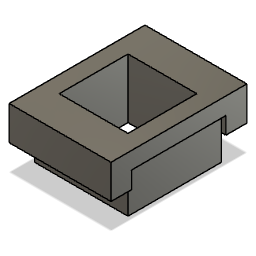
switch_holder (Autodesk Fusion 360 design; units mm, degrees)
Autodesk Fusion 360 part; units mm, degrees
note: some values were not read from the file. Set by a fixed rule: which sketch regions a step uses.
sketch "Sketch1" plane through (0, 0, 0) normal (0, 1, 0) x (1, 0, 0)
  line L0 (5.5, 5.5) -> (-5.5, 5.5)
  line L1 (-5.5, 5.5) -> (-5.5, -5.5)
  line L2 (-5.5, -5.5) -> (5.5, -5.5)
  line L3 (5.5, -5.5) -> (5.5, 5.5)
  line L4 (5.5, 5.5) -> (-5.5, -5.5) construction
  line L5 (-5.5, 5.5) -> (5.5, -5.5) construction
  dimension "d1" = 11
  dimension "d2" = 11
  constraint horizontal L0
  constraint perpendicular L0 L1
  constraint parallel L0 L2
  constraint parallel L1 L3
  constraint coincident L4 origin
  constraint coincident L5 origin
  measures "d1" distance of L1.end L2.end
  measures "d2" distance of L0.end L1.end
extrude "Extrude1" add sketch "Sketch1" along normal blind 5
sketch "Sketch2" plane through (0, 5, 0) normal (0, 1, 0) x (-1, 0, 0)
  line L0 (-5.5, 5.5) -> (-5.5, -5.5)
  line L1 (-5.5, -5.5) -> (5.5, -5.5)
  line L2 (5.5, -5.5) -> (5.5, 5.5)
  line L3 (5.5, 5.5) -> (-5.5, 5.5)
  line L4 (-4.05, -4.05) -> (4.05, -4.05)
  line L5 (4.05, -4.05) -> (4.05, 4.05)
  line L6 (4.05, 4.05) -> (-4.05, 4.05)
  line L7 (-4.05, 4.05) -> (-4.05, -4.05)
  line L8 (-4.05, -4.05) -> (4.05, 4.05) construction
  line L9 (4.05, -4.05) -> (-4.05, 4.05) construction
  dimension "d5" = 8.1
  dimension "d6" = 8.1
  constraint horizontal L4
  constraint perpendicular L4 L5
  constraint parallel L4 L6
  constraint parallel L5 L7
  constraint coincident L8 origin
  constraint coincident L9 origin
  measures "d5" distance of L5.end L6.end
  measures "d6" distance of L4.end L5.end
extrude "Extrude2" cut sketch "Sketch2" against normal blind 5 contours L4 L5 L6 L7
sketch "Sketch3" plane through (0, 5, 0) normal (0, 1, 0) x (-1, 0, 0)
  line L0 (4.05, -4.05) -> (-4.05, -4.05)
  line L1 (-4.05, -4.05) -> (-4.05, 4.05)
  line L2 (-4.05, 4.05) -> (4.05, 4.05)
  line L3 (4.05, 4.05) -> (4.05, -4.05)
  line L4 (-5.5, 5.5) -> (-5.5, -5.5)
  line L5 (-5.5, -5.5) -> (5.5, -5.5)
  line L6 (5.5, -5.5) -> (5.5, 5.5)
  line L7 (5.5, 5.5) -> (-5.5, 5.5)
  line L8 (-6, -8) -> (6, -8)
  line L9 (6, -8) -> (6, 8)
  line L10 (6, 8) -> (-6, 8)
  line L11 (-6, 8) -> (-6, -8)
  line L12 (-6, -8) -> (6, 8) construction
  line L13 (6, -8) -> (-6, 8) construction
  dimension "d9" = 12
  dimension "d10" = 16
  constraint horizontal L8
  constraint perpendicular L8 L9
  constraint parallel L8 L10
  constraint parallel L9 L11
  constraint coincident L12 origin
  constraint coincident L13 origin
  measures "d9" distance of L9.end L10.end
  measures "d10" distance of L8.end L9.end
extrude "Extrude3" add sketch "Sketch3" along normal blind 2 contours L4 L5 L6 L7 | L8 L9 L10 L11
sketch "Sketch4" plane through (0, 5, 0) normal (0, -1, 0) x (1, 0, 0)
  line L0 (6, -8) -> (6, 8)
  line L1 (6, 8) -> (-6, 8)
  line L2 (-6, 8) -> (-6, -8)
  line L3 (-6, -8) -> (6, -8)
  line L4 (-5.5, 5.5) -> (5.5, 5.5)
  line L5 (5.5, 5.5) -> (5.5, -5.5)
  line L6 (5.5, -5.5) -> (-5.5, -5.5)
  line L7 (-5.5, -5.5) -> (-5.5, 5.5)
  line L8 (6, 8) -> (-6, 8)
  line L9 (-6, 8) -> (-6, 5.5772)
  line L10 (-6, 5.5772) -> (6, 5.5772)
  line L11 (6, 5.5772) -> (6, 8)
  line L12 (6, -8) -> (-6, -8)
  line L13 (-6, -8) -> (-6, -5.5258)
  line L14 (-6, -5.5258) -> (6, -5.5258)
  line L15 (6, -5.5258) -> (6, -8)
  constraint horizontal L8
  constraint vertical L9
  constraint horizontal L10
  constraint vertical L11
  constraint coincident L2 L9.end
  constraint coincident L0.end L1.start
  constraint horizontal L12
  constraint vertical L13
  constraint horizontal L14
  constraint vertical L15
  constraint coincident L2 L13.end
  constraint coincident L0.start L3.end
extrude "Extrude4" add sketch "Sketch4" along normal blind 2 contours L0 L2 L3 L12 L13 L14 L15 | L0 L1 L2 L8 L9 L10 L11
